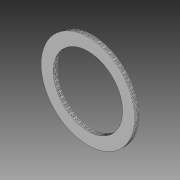
# Autodesk Inventor part: AXK4060 thrust bearing
Saved by Autodesk Inventor 2020 (Build 240168000, 168)
## iProperties
Created: 2021-04-24
Part Number: AXK4060 thrust bearing
Material: Generic
Document SubType Name: Modeling
Designer: DDeGo
Density: 1 g/cm^3
Appearance: Default
Author: DDeGo
Autodesk Inventor part; units mm, degrees
ref_plane "YZ Plane" through (0, 0, 0) normal (1, 0, 0) x (0, 1, 0)
ref_plane "XZ Plane" through (0, 0, 0) normal (0, 1, 0) x (-1, 0, 0)
ref_plane "XY Plane" through (0, 0, 0) normal (0, 0, 1) x (1, 0, 0)
sketch "Sketch1" plane through (0, 0, 0) normal (0, 0, 1) x (1, 0, 0)
  circle A0 centre (0, 0) radius 50
  circle A1 centre (0, 0) radius 67.5
  dimension "d0" = 100
  dimension "d1" = 135
  constraints: 2 centre point, 2 coincident
  measures "d0" diameter of A0
  measures "d1" diameter of A1
extrude "Extrusion1" add sketch "Sketch1" along normal mid plane 1
sketch "Sketch2" plane through (0, 0, 0) normal (0, 0, 1) x (1, 0, 0)
  line L0 (0, 0) -> (-59.0774, 0) construction
  circle A0 centre (0, 0) radius 50 construction
  line L1 (-50, 0) -> (-67.4704, 0)
  line L2 (-67.4704, 0) -> (-67.4704, -2)
  line L3 (-67.4704, -2) -> (-50, -2)
  line L4 (-50, -2) -> (-50, 0)
  circle A1 centre (0, 0) radius 67.5 construction
  dimension "d4" = 2
  constraints: 10 end point, 2 horizontal, 2 parallel, 1 horizontal alignment, 1 perpendicular, 1 point on line, 3 other
  measures "d4" distance between parallel lines of L3 L0
revolve "Revolution1" add sketch "Sketch2" angle 360 about axis through (0, 0, 0) along (-1, 0, 0)
pattern_circular "Circular Pattern1" count 50 over 360 about axis through (0, 0, -10) along (0, 0, 1) of "Revolution1"
sketch "Sketch3" plane through (0, 0, 0) normal (0, 1, 0) x (-1, 0, 0)
  line L0 (50, 2) -> (67.4704, 2) projected
  line L1 (67.4704, 2) -> (50, 2)
  line L2 (50, 2) -> (50, 3)
  line L3 (50, 3) -> (67.4704, 3)
  line L4 (67.4704, 3) -> (67.4704, 2)
  line L5 (67.4704, -2) -> (67.4704, -0.5) projected
  line L6 (67.4704, -2) -> (50, -2)
  line L7 (50, -2) -> (50, -3)
  line L8 (50, -3) -> (67.4704, -3)
  line L9 (67.4704, -3) -> (67.4704, -2)
  line L10 (50, -2) -> (50, -0.5) projected
  line L11 (67.4704, 0.5) -> (67.4704, 2) projected
  line L12 (0, 0) -> (0, 25.6351) construction
  dimension "d9" = 1
  dimension "d10" = 1
  constraints: 18 end point, 4 parallel, 4 point on line, 2 horizontal, 2 perpendicular, 1 vertical
  measures "d9" distance of L3.end L1.start
  measures "d10" distance of L8.end L5.start
revolve "Revolution2" add sketch "Sketch3" angle 360 about axis through (0, 0, 0) along (0, 0, 1)
body "Solid1"
